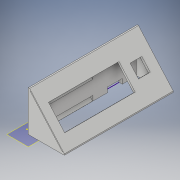
# Autodesk Inventor part: Suport - pantalla i potenciometre
Saved by Autodesk Inventor 2019 (Build 230136000, 136)
## iProperties
Created: 2018-08-18
Part Number: Suport - pantalla i potenciometre
Material: Genérico
Document SubType Name: Modeling
Designer: Albert Garangou Culebras
Density: 1 g/cm^3
Appearance: Valor por defecto
Author: Albert Garangou Culebras
Autodesk Inventor part; units mm, degrees
ref_plane "YZ Plane" through (0, 0, 0) normal (1, 0, 0) x (0, 1, 0)
ref_plane "XZ Plane" through (0, 0, 0) normal (0, 1, 0) x (-1, 0, 0)
ref_plane "XY Plane" through (0, 0, 0) normal (0, 0, 1) x (1, 0, 0)
sketch "Boceto3" plane through (0, 0, 0) normal (0, 0, 1) x (1, 0, 0)
  line L0 (40, 0) -> (37, 0)
  line L1 (0, 0) -> (0, 45)
  line L2 (0, 45) -> (3, 45)
  line L3 (40, 0) -> (40, 3)
  line L4 (40, 3) -> (3, 45)
  line L5 (0, 0) -> (40, 0)
  dimension "d3" = 3
  dimension "d4" = 45
  dimension "d5" = 3
  dimension "d6" = 3
  constraints: 12 end point, 2 horizontal, 2 vertical, 1 perpendicular
  measures "d3" distance of L0.start L0.end
  measures "d4" distance of L1.start L1.end
  measures "d5" distance of L1.end L2.end
  measures "d6" distance of L0.start L3.end
extrude "Extrusión1" add sketch "Boceto3" against normal blind 98.2
sketch "Boceto4" plane through (0, 0, 0) normal (0, 0, 1) x (1, 0, 0)
  line L0 (3.315362, 41.620064) -> (2, 43)
  line L1 (3.315362, 41.620064) -> (38, 2)
  line L2 (38, 2) -> (2, 2)
  line L3 (2, 2) -> (2, 43)
  point P0 (0, 45)
  constraints: 8 end point, 1 horizontal
extrude "Extrusión2" cut sketch "Boceto4" against normal blind 210.55
sketch "Boceto6" plane through (0, 0, 0) normal (0, 0, 1) x (1, 0, 0)
  line L0 (1.039471, 0.999221) -> (39.039471, 0.999221)
  line L1 (39.039471, 1.000307) -> (39.039471, 1.999307)
  line L2 (39.039471, 0.999221) -> (39.039471, 1.999307)
  line L3 (39.039471, 1.999307) -> (3, 44.000307)
  line L4 (2.880008, 44.000307) -> (1.000008, 44.000307)
  line L5 (3, 44.000307) -> (1.000008, 44.000307)
  line L6 (1.000008, 1.000307) -> (39.039471, 1.000307)
  line L7 (1.000008, 44.000307) -> (1.000008, 1.000307)
  point P0 (0, 0)
  constraints: 10 end point, 2 perpendicular, 1 horizontal, 1 parallel
extrude "Extrusión3" add sketch "Boceto6" against normal blind 2
sketch "Boceto7" plane through (0, 0, -98.2) normal (0, 0, -1) x (-1, 0, 0)
  line L0 (-1.000008, 1.000307) -> (-39.039471, 1.000307)
  line L1 (-1.000008, 1.000307) -> (-39.039471, 1.000307)
  line L2 (-39.039471, 1.000307) -> (-39.039471, 2)
  line L3 (-39.039471, 1.999307) -> (-2.880008, 44.000307)
  line L4 (-39.039471, 2) -> (-2.880008, 44.000307)
  line L5 (-2.880008, 44.000307) -> (-1.000008, 44.000307)
  line L6 (-1.000008, 44.000307) -> (-1.000008, 1.000307)
  line L7 (-2.880008, 44.000307) -> (6.906678, 55.367839)
  line L8 (6.906678, 55.367839) -> (10.168907, 59.157016)
  line L9 (10.168907, 59.157016) -> (10.168907, 0)
  line L10 (10.168907, 0) -> (0, 0)
  dimension "d68" = 15
  dimension "d70" = 5
  constraints: 17 end point, 2 perpendicular, 2 vertical, 1 collinear
  measures "d68" distance of L3.end L7.end
  measures "d70" distance of L7.end L8.end
extrude "Extrusión4" add sketch "Boceto7" against normal blind 2
sketch "Boceto10" plane through (0, 0, -96.2) normal (0, 0, 1) x (1, 0, 0)
  line L0 (20.169084, 1.000307) -> (21.669084, 1.000307)
  line L1 (39.039471, 1.000307) -> (1.000008, 1.000307)
  line L2 (21.669084, 1.000307) -> (21.669084, 22.175869)
  line L3 (2.880008, 44.000307) -> (39.039471, 1.999307)
  line L4 (21.669084, 22.175869) -> (20.169084, 23.918193)
  line L5 (20.169084, 23.918193) -> (20.169084, 1.000307)
  point P0 (0, 0)
  dimension "d49" = 1.5
  constraints: 8 end point, 2 point on line, 1 collinear, 1 parallel, 1 vertical
  measures "d49" distance of L0.start L0.end
extrude "Extrusión7" add sketch "Boceto10" along normal blind 96
sketch "Boceto15" plane through (0, 0, -98.2) normal (0, 0, -1) x (-1, 0, 0)
  line L0 (-3, 45) -> (-40, 3)
  line L1 (-20.392682, 25.256955) -> (-7.172072, 40.264135)
  line L2 (-7.172072, 40.264135) -> (-7.172072, 0)
  line L3 (-20.169084, 1.000307) -> (-1.000008, 1.000307)
  line L4 (-7.172072, 40.264135) -> (-3, 45)
  line L5 (0, 45) -> (-3, 45)
  line L6 (0, 0) -> (0, 45)
  line L7 (0, 45) -> (0, 0)
  line L8 (0, 0) -> (-7.172072, 0)
  line L9 (-40, 0) -> (0, 0)
  dimension "d71" = 20
  constraints: 12 end point, 3 collinear, 2 point on line, 1 horizontal, 1 perpendicular
  measures "d71" distance of L1.start L1.end
extrude "Extrusión9" cut sketch "Boceto15" against normal blind 617.4
sketch "Boceto16" plane through (0, 0, -96.2) normal (0, 0, 1) x (1, 0, 0)
  line L0 (7.172072, 0.999997) -> (8.672072, 1.000307)
  line L1 (20.169084, 1.000307) -> (7.172072, 1.000307)
  line L2 (8.672072, 1.000307) -> (8.672072, 37.27254)
  line L3 (7.172072, 39.014864) -> (20.169084, 23.918193)
  line L4 (8.672072, 37.27254) -> (7.172072, 39.014864)
  line L5 (7.172072, 39.014864) -> (7.172072, 0.999997)
  point P0 (0, 0)
  dimension "d74" = 1.5
  constraints: 8 end point, 1 collinear, 1 parallel, 1 perpendicular, 1 point on line
  measures "d74" distance of L0.start L0.end
extrude "Extrusión10" add sketch "Boceto16" along normal blind 95.4
sketch "Boceto17" plane through (0, 0, 0) normal (0, 0, 1) x (1, 0, 0)
  line L0 (20.169084, 1.000307) -> (8.672072, 1.000307)
  line L1 (8.672072, 35.501126) -> (8.672072, 2)
  line L2 (8.672072, 1.000307) -> (8.672072, 37.27254)
  line L3 (39.039471, 1.999307) -> (21.669084, 22.175869)
  line L4 (8.672072, 37.27254) -> (39.039471, 1.999307)
  line L5 (39.039471, 1.999307) -> (39.039471, 1.000307)
  line L6 (39.039471, 1.000307) -> (8.672072, 1.000307)
  line L7 (40, 0) -> (7.172072, 0)
  point P0 (0, 0)
  constraints: 8 end point, 2 collinear, 2 parallel
extrude "Extrusión11" cut sketch "Boceto17" against normal blind 235.6
sketch "Boceto21" plane through (40, 3, 0) normal (0.750359, 0.6610305, 0) x (0, 0, -1)
  line L0 (5, 24.190145) -> (5, 36.190145)
  line L1 (5, 36.190145) -> (5, 12.190145)
  line L2 (76, 36.190145) -> (5, 36.190145)
  line L3 (85, 24.190145) -> (85, 18.190145)
  line L4 (85, 18.190145) -> (91, 18.190145)
  line L5 (91, 18.190145) -> (97, 18.190145)
  line L6 (97, 18.190145) -> (97, 30.190145)
  line L7 (97, 30.190145) -> (85, 30.190145)
  line L8 (85, 30.190145) -> (85, 24.190145)
  line L9 (76, 24.190145) -> (81, 24.190145)
  line L10 (81, 24.190145) -> (85, 24.190145)
  line L11 (76, 36.190145) -> (77, 36.190145)
  line L12 (77, 36.190145) -> (77, 12.190145)
  line L13 (77, 12.190145) -> (76, 12.190145)
  line L14 (77, 12.190145) -> (77, 11.190145)
  line L15 (77, 11.190145) -> (5, 11.190145)
  line L16 (5, 11.190145) -> (5, 12.190145)
  point P0 (0, 24.190145)
  dimension "d114" = 5
  dimension "d176" = 1
  dimension "d177" = 1
  constraints: 34 end point, 7 perpendicular, 3 horizontal, 3 point on line, 1 vertical
  measures "d114" distance of L9.end L9.start
  measures "d176" distance of L2.start L11.end
  measures "d177" distance of L12.end L14.end
extrude "Extrusión13" cut sketch "Boceto21" against normal blind 1.5
sketch "Boceto22" plane through (0, 0, 0) normal (0, 0, 1) x (1, 0, 0)
  line L0 (8.672072, 1.000307) -> (39.039471, 1.000307)
  line L1 (8.672072, 1.000307) -> (39.039471, 1.000307)
  line L2 (39.039471, 1.000307) -> (39.039471, 2)
  line L3 (39.039471, 2) -> (8.672072, 37)
  line L4 (8.672072, 37.27254) -> (8.672072, 1.000307)
  line L5 (8.672072, 37) -> (8.672072, 1.000307)
  line L6 (7.172072, 0) -> (7.172072, 40.264135)
  line L7 (7.172072, 40.264135) -> (7.172072, 0)
  line L8 (40, 3) -> (40, 0)
  line L9 (7.172072, 0) -> (40, 0)
  line L10 (40, 0) -> (40, 3)
  line L11 (40, 3) -> (7.172072, 40.264135)
  line L12 (7.172072, 40.264135) -> (40, 3)
  point P0 (0, 0)
  constraints: 16 end point, 3 collinear, 3 perpendicular, 1 horizontal
extrude "Extrusión14" add sketch "Boceto22" along normal blind 2
sketch "Boceto24" plane through (0, 0, 2) normal (0, 0, 1) x (1, 0, 0)
  line L0 (8.672072, 1.000307) -> (8.672072, 37)
  line L1 (39.039471, 1.000307) -> (8.672072, 1.000307)
  line L2 (8.672072, 1.000307) -> (39.039471, 1.000307)
  line L3 (39.039471, 1.000307) -> (39.039471, 2)
  line L4 (39.039471, 2) -> (8.672072, 37)
  line L5 (8.672072, 37) -> (8.672072, 1.000307)
  point P0 (0, 0)
  constraints: 8 end point, 1 collinear, 1 parallel, 1 perpendicular
extrude "Extrusión15" add sketch "Boceto24" against normal blind 2
sketch "Boceto25" plane through (0, 0, -98.2) normal (0, 0, -1) x (-1, 0, 0)
  line L0 (-8.672072, 1.000307) -> (-8.672072, 37.27254)
  line L1 (-8.672072, 1.000307) -> (-8.672072, 37.27254)
  line L2 (-8.672072, 37.27254) -> (-39, 2)
  line L3 (-39, 2) -> (-39, 1.000307)
  line L4 (-39, 1.000307) -> (-8.672072, 1.000307)
  line L5 (-7.172072, 0) -> (-40, 0)
  line L6 (-7.172072, 40) -> (-7.172072, 0)
  line L7 (-40, 0) -> (-7.172072, 0)
  line L8 (-40, 0) -> (-40, 2.859817)
  line L9 (-7.172072, 0) -> (-7.172072, 40.264135)
  line L10 (-40, 2.859817) -> (-7.172072, 40.264135)
  point P0 (0, 0)
  constraints: 16 end point, 2 parallel, 2 vertical, 1 collinear, 1 perpendicular
extrude "Extrusión16" add sketch "Boceto25" along normal blind 7
sketch "Boceto27" plane through (0, 0, -105.2) normal (0, 0, -1) x (-1, 0, 0)
  line L0 (-8.672072, 1.000307) -> (-39.039471, 1.000307)
  line L1 (-8.672072, 1.000307) -> (-39.039471, 1.000307)
  line L2 (-39.039471, 1.000307) -> (-39.039471, 1.999307)
  line L3 (-8.672072, 1.000307) -> (-8.672072, 37.27254)
  line L4 (-39.039471, 1.999307) -> (-8.672072, 37.27254)
  line L5 (-8.672072, 37.27254) -> (-8.672072, 1.000307)
  point P0 (0, 0)
  constraints: 8 end point, 2 collinear, 1 perpendicular
extrude "Extrusión17" add sketch "Boceto27" against normal blind 2
sketch "Boceto28" plane through (7.172072, 0, 2) normal (0, -1, 0) x (1, 0, 0)
  line L0 (0, 0) -> (0, -107.2)
  line L1 (32.827928, 0) -> (32.827928, -107.2)
  line L2 (0, 0) -> (32.827928, 0)
  line L3 (32.827928, 0) -> (32.827928, -107.2)
  line L4 (32.827928, -107.2) -> (0, -107.2)
  line L5 (0, -107.2) -> (0, 0)
  point P0 (-7.172072, -2)
  constraints: 8 end point, 2 parallel, 1 horizontal, 1 perpendicular
extrude "Extrusión18" add sketch "Boceto28" along normal blind 2
sketch "Boceto29" plane through (7.172072, 40.264135, -98.2) normal (-1, 0, 0) x (0, 0, 1)
  line L0 (0, 0) -> (-7, 0)
  line L1 (100.2, -37.264135) -> (100.2, -42.264135)
  line L2 (-7, 0) -> (100.2, 0)
  line L3 (100.2, 0) -> (100.2, -42.264135)
  line L4 (100.2, -42.264135) -> (-7, -42.264135)
  line L5 (-7, -42.264135) -> (-7, 0)
  point P0 (98.2, -40.264135)
  constraints: 8 end point, 2 parallel, 1 horizontal, 1 perpendicular
extrude "Extrusión19" add sketch "Boceto29" along normal blind 2
sketch "Boceto30" plane through (0, 0, -105.2) normal (0, 0, -1) x (-1, 0, 0)
  line L0 (-7.172072, 40.264135) -> (-5.172072, 40.264135)
  line L1 (-5.172072, 40.264135) -> (-5.172072, -2)
  line L2 (-5.172072, 40.264135) -> (-5.172072, -2)
  line L3 (-40, -2) -> (-5.172072, -2)
  line L4 (-5.172072, -2) -> (-40, -2)
  line L5 (-40, 2.859817) -> (-40, -2)
  line L6 (-40, -2) -> (-40, 2.859817)
  line L7 (-40, 2.859817) -> (-7.172072, 40.264135)
  line L8 (-7.172072, 40.264135) -> (-5.172072, 40.264135)
  point P0 (0, 0)
  constraints: 12 end point, 3 collinear, 1 horizontal, 1 perpendicular
extrude "Extrusión20" add sketch "Boceto30" along normal blind 2
sketch "Boceto31" plane through (0, 0, 2) normal (0, 0, 1) x (1, 0, 0)
  line L0 (5.172072, -2) -> (5.172072, 40.264135)
  line L1 (5.172072, 40.26431) -> (5.172072, -2)
  line L2 (40, -2) -> (5.172072, -2)
  line L3 (5.172072, -2) -> (40, -2)
  line L4 (40, 2.859817) -> (40, -2)
  line L5 (40, -2) -> (40, 2.859817)
  line L6 (40, 2.859817) -> (7.172072, 40.264135)
  line L7 (7.172072, 40.264135) -> (40, 2.859817)
  line L8 (7.172072, 40.264135) -> (5.172072, 40.264135)
  point P0 (0, 0)
  constraints: 11 end point, 3 collinear, 1 horizontal
extrude "Extrusión21" add sketch "Boceto31" along normal blind 2
sketch "Boceto32" plane through (40, 3, 2) normal (0.750359, 0.6610305, 0) x (0, 0, -1)
  line L0 (-2, 49.661742) -> (-2, 0)
  line L1 (-2, 0) -> (109.2, 0)
  line L2 (109.2, -3.751795) -> (109.2, 19.270529)
  line L3 (100.2, -0.105188) -> (109.2, -0.105188)
  line L4 (109.2, 49.661742) -> (109.2, -0.105188)
  line L5 (109.2, 49.661742) -> (-2, 49.661742)
  line L6 (-2, 50.983803) -> (-2, 19.270529)
  line L7 (7, 11.190145) -> (7, 36.190145)
  line L8 (7, 36.190145) -> (7, 12.190145)
  line L9 (78, 36.190145) -> (7, 36.190145)
  line L10 (87, 30.190145) -> (99, 30.190145)
  line L11 (87, 18.190145) -> (87, 30.190145)
  line L12 (87, 30.190145) -> (87, 18.190145)
  line L13 (99, 30.190145) -> (99, 18.190145)
  line L14 (87, 18.190145) -> (99, 18.190145)
  line L15 (99, 18.190145) -> (99, 30.190145)
  line L16 (100.2, 49.661742) -> (109.2, 49.661742)
  line L17 (109.2, 49.661742) -> (109.2, -0.105188)
  line L18 (-2, -3.751795) -> (-2, -0.105188)
  line L19 (109.2, -0.105188) -> (-2, -0.105188)
  line L20 (-2, -0.105188) -> (-2, 49.661742)
  line L21 (109.2, 49.661742) -> (-2, 49.661742)
  line L22 (87, 30.190145) -> (99, 30.190145)
  line L23 (7, 12.190145) -> (7, 11.190145)
  line L24 (7, 11.190145) -> (79, 11.190145)
  line L25 (79, 11.190145) -> (79, 36.190145)
  line L26 (79, 36.190145) -> (78, 36.190145)
  point P0 (2, 24.190145)
  dimension "d174" = 1
  dimension "d175" = 72
  constraints: 36 end point, 7 collinear, 6 perpendicular, 2 point on line, 2 vertical, 1 horizontal
  measures "d174" distance of L8.end L7.start
  measures "d175" distance of L7.start L24.end
extrude "Extrusión22" add sketch "Boceto32" along normal blind 1
sketch "Boceto33" plane through (40.750359, 3.661031, 2) normal (0.750359, 0.6610305, 0) x (0, 0, -1)
  line L0 (87, 30.190145) -> (87, 18.190145)
  line L1 (87, 30.190145) -> (99, 30.190145)
  line L2 (87, 30.190145) -> (99, 30.190145)
  line L3 (99, 30.190145) -> (99, 18.133841)
  line L4 (100.2, -0.105188) -> (100.2, 49.661742)
  line L5 (99, 18.133841) -> (87, 18.133841)
  line L6 (87, 30.190145) -> (87, 34.190145)
  line L7 (87, 34.190145) -> (83, 34.190145)
  line L8 (99, 18.190145) -> (99, 14.190145)
  line L9 (99, 14.190145) -> (103, 14.190145)
  line L10 (83, 34.190145) -> (103, 34.190145)
  line L11 (103, 34.190145) -> (103, 14.190145)
  line L12 (103, 14.190145) -> (83, 14.190145)
  line L13 (83, 14.190145) -> (83, 34.190145)
  point P0 (2, 24.190145)
  dimension "d126" = 4
  dimension "d127" = 4
  dimension "d129" = 4
  dimension "d130" = 4
  constraints: 22 end point, 4 perpendicular, 3 parallel, 2 horizontal, 2 vertical
  measures "d126" distance of L0.start L6.end
  measures "d127" distance of L6.end L7.end
  measures "d129" distance of L8.start L8.end
  measures "d130" distance of L8.end L9.end
extrude "Extrusión23" add sketch "Boceto33" against normal blind 2.5
sketch "Boceto34" plane through (40.750359, 3.661031, 2) normal (0.750359, 0.6610305, 0) x (0, 0, -1)
  line L0 (99, 18.190145) -> (99, 30.190145)
  line L1 (99, 18.190145) -> (87, 18.190145)
  line L2 (87, 18.190145) -> (87, 30.190145)
  line L3 (99, 30.190145) -> (99, 18.190145)
  line L4 (99, 30.190145) -> (99, 18.190145)
  line L5 (87, 18.190145) -> (99, 18.190145)
  line L6 (99, 30.190145) -> (99, 31.190145)
  line L7 (99, 31.190145) -> (87, 31.190145)
  line L8 (87, 31.190145) -> (87, 30.190145)
  point P0 (2, 24.190145)
  point P1 (83, 34.190145)
  dimension "d173" = 1
  constraints: 18 end point, 3 perpendicular, 1 collinear, 1 point on line
  measures "d173" distance of L0.end L6.end
extrude "Extrusión24" cut sketch "Boceto34" against normal blind 6
sketch "Boceto35" plane through (40.069532, 2.921072, 4) normal (0, 0, 1) x (0.750359, 0.6610305, 0)
  line L0 (0, 49.76693) -> (1, 49.76693)
  line L1 (1, 49.76693) -> (0, 49.76693)
  line L2 (0, 49.76693) -> (0, 0)
  line L3 (0, 0) -> (1, 0)
  line L4 (0, 0) -> (1, 0)
  line L5 (1, 0) -> (1, 49.76693)
  point P0 (-31.997451, 24.295332)
  constraints: 8 end point, 3 perpendicular, 1 horizontal
extrude "Extrusión25" cut sketch "Boceto35" against normal blind 0.0001
sketch "Boceto36" plane through (0, 0, 4) normal (0, 0, 1) x (1, 0, 0)
  line L0 (5.172072, 40.264135) -> (7.172072, 40.264135)
  line L1 (7.172072, 40.264135) -> (40, 2.859817)
  line L2 (5.172072, 40.264135) -> (7.172072, 40.264135)
  line L3 (7.172072, 40.264135) -> (7.922431, 40.925165)
  line L4 (7.172072, 40.264135) -> (7.922431, 40.925165)
  line L5 (7.922431, 40.925165) -> (6.60037, 42.425883)
  line L6 (6.60037, 42.425883) -> (5.172072, 42.425883)
  line L7 (5.172072, -2) -> (5.172072, 40.264135)
  line L8 (5.172072, 42.425883) -> (5.172072, 40.264135)
  point P0 (0, 0)
  dimension "d140" = 2
  constraints: 10 end point, 2 perpendicular, 1 collinear, 1 horizontal, 1 parallel
  measures "d140" distance of L3.end L5.end
extrude "Extrusión26" add sketch "Boceto36" against normal blind 111.22
sketch "Boceto37" plane through (0, 0, 4) normal (0, 0, 1) x (1, 0, 0)
  line L0 (40.069532, 2.921072) -> (7.172072, 40.264135)
  line L1 (40.069532, 2.921072) -> (39.994609, 2.855068)
  line L2 (39.994609, 2.855068) -> (7.13461, 40.231133)
  line L3 (7.172072, 40.264135) -> (7.922431, 40.925165)
  line L4 (7.13461, 40.231133) -> (7.922431, 40.925165)
  line L5 (7.922431, 40.925165) -> (40.069532, 2.921072)
  point P0 (0, 0)
  constraints: 8 end point, 1 collinear, 1 perpendicular
extrude "Extrusión27" add sketch "Boceto37" against normal blind 2 contours L1 L2 L4 L0
sketch "Boceto38" plane through (0, 0, 4) normal (0, 0, 1) x (1, 0, 0)
  line L0 (40, 2.859817) -> (40, -2)
  line L1 (40, -2) -> (40, 2.859817)
  line L2 (40.069532, 2.921072) -> (40.819891, 3.582102)
  line L3 (40, 2.859817) -> (40.819891, 3.582102)
  line L4 (40, -2) -> (42, -2)
  line L5 (42, -2) -> (42, 2.242519)
  line L6 (42, 2.242519) -> (40.819891, 3.582102)
  point P0 (0, 0)
  constraints: 10 end point, 2 collinear, 1 perpendicular
extrude "Extrusión28" add sketch "Boceto38" against normal blind 111.25
sketch "Boceto39" plane through (0, 0, -107.2) normal (0, 0, -1) x (-1, 0, 0)
  line L0 (-40.069532, 2.921072) -> (-40.819891, 3.582102)
  line L1 (-40.069532, 2.921072) -> (-40, 2.859817)
  line L2 (-40.069532, 2.921072) -> (-7.172072, 40.264135)
  line L3 (-40, 2.859817) -> (-7.172072, 40.264135)
  line L4 (-7.172072, 40.264135) -> (-40.069532, 2.921072)
  line L5 (-40.069532, 2.921072) -> (-40, 2.859817)
  point P0 (0, 0)
  constraints: 8 end point, 2 collinear, 1 perpendicular
extrude "Extrusión29" add sketch "Boceto39" against normal blind 2
sketch "Boceto40" plane through (7.172072, -2, 2) normal (0, -1, 0) x (1, 0, 0)
  line L0 (7.786838, -16.048701) -> (16.767817, -16.048701) construction
  line L1 (16.767817, -16.048701) -> (16.767817, -19.096701) construction
  line L2 (16.767817, -19.096701) -> (7.786838, -19.096701) construction
  line L3 (7.786838, -19.096701) -> (7.786838, -16.048701) construction
  spline S0 degree 2 poles (12.542267, -20.275201) (12.542267, -20.729982) (12.196238, -21.426984) (11.909528, -21.654374) knots 0 0 0 1 2 2 2
  spline S1 degree 2 poles (11.909528, -21.654374) (11.563499, -21.921311) (10.777519, -22.148702) (10.154666, -22.148702) knots 0 0 0 1 2 2 2
  line L4 (10.154666, -22.148702) -> (8.404747, -22.148702)
  line L5 (8.404747, -22.148702) -> (8.404747, -16.048701)
  line L6 (8.404747, -16.048701) -> (10.021198, -16.048701)
  spline S2 degree 2 poles (10.021198, -16.048701) (10.67371, -16.048701) (11.326222, -16.132737) (11.622818, -16.295865) knots 0 0 0 1 2 2 2
  spline S3 degree 2 poles (11.622818, -16.295865) (11.954018, -16.46888) (12.255558, -17.037356) (12.255558, -17.422932) knots 0 0 0 1 2 2 2
  spline S4 degree 2 poles (12.255558, -17.422932) (12.255558, -17.852996) (11.800776, -18.535168) (11.400371, -18.727956) knots 0 0 0 1 2 2 2
  line L7 (11.400371, -18.727956) -> (11.400371, -18.757616)
  spline S5 degree 2 poles (11.400371, -18.757616) (11.944131, -18.905914) (12.542267, -19.691894) (12.542267, -20.275201) knots 0 0 0 1 2 2 2
  spline S6 degree 2 poles (11.696968, -20.309804) (11.696968, -19.963774) (11.499237, -19.51888) (11.20264, -19.360695) knots 0 0 0 1 2 2 2
  spline S7 degree 2 poles (11.20264, -19.360695) (11.009852, -19.26183) (10.555071, -19.20251) (10.134893, -19.20251) knots 0 0 0 1 2 2 2
  line L8 (10.134893, -19.20251) -> (9.215444, -19.20251)
  line L9 (9.215444, -19.20251) -> (9.215444, -21.456643)
  line L10 (9.215444, -21.456643) -> (9.872899, -21.456643)
  spline S8 degree 2 poles (9.872899, -21.456643) (10.406773, -21.456643) (11.019739, -21.357778) (11.257016, -21.199593) knots 0 0 0 1 2 2 2
  spline S9 degree 2 poles (11.257016, -21.199593) (11.484407, -21.036465) (11.696968, -20.631116) (11.696968, -20.309804) knots 0 0 0 1 2 2 2
  spline S10 degree 2 poles (11.410258, -17.536627) (11.410258, -17.319123) (11.261959, -16.992867) (11.098831, -16.898945) knots 0 0 0 1 2 2 2
  spline S11 degree 2 poles (11.098831, -16.898945) (10.9011, -16.790193) (10.421603, -16.74076) (9.991538, -16.74076) knots 0 0 0 1 2 2 2
  line L11 (9.991538, -16.74076) -> (9.215444, -16.74076)
  line L12 (9.215444, -16.74076) -> (9.215444, -18.525282)
  line L13 (9.215444, -18.525282) -> (10.134893, -18.525282)
  spline S12 degree 2 poles (10.134893, -18.525282) (10.515525, -18.525282) (10.876384, -18.446189) (11.069172, -18.322607) knots 0 0 0 1 2 2 2
  spline S13 degree 2 poles (11.069172, -18.322607) (11.257016, -18.203969) (11.410258, -17.823337) (11.410258, -17.536627) knots 0 0 0 1 2 2 2
  line L14 (12.690566, -22.148702) -> (14.746968, -16.048701)
  line L15 (14.746968, -16.048701) -> (15.745509, -16.048701)
  line L16 (15.745509, -16.048701) -> (17.801911, -22.148702)
  line L17 (17.801911, -22.148702) -> (16.946725, -22.148702)
  line L18 (16.946725, -22.148702) -> (16.393078, -20.443272)
  line L19 (16.393078, -20.443272) -> (14.064796, -20.443272)
  line L20 (14.064796, -20.443272) -> (13.511149, -22.148702)
  line L21 (13.511149, -22.148702) -> (12.690566, -22.148702)
  line L22 (16.170631, -19.751214) -> (15.226465, -16.879171)
  line L23 (15.226465, -16.879171) -> (14.287243, -19.751214)
  line L24 (14.287243, -19.751214) -> (16.170631, -19.751214)
  line L25 (20.505882, -22.148702) -> (18.142997, -22.148702)
  line L26 (18.142997, -22.148702) -> (18.142997, -21.525849)
  line L27 (18.142997, -21.525849) -> (18.919091, -21.525849)
  line L28 (18.919091, -21.525849) -> (18.919091, -16.671554)
  line L29 (18.919091, -16.671554) -> (18.142997, -16.671554)
  line L30 (18.142997, -16.671554) -> (18.142997, -16.048701)
  line L31 (18.142997, -16.048701) -> (20.505882, -16.048701)
  line L32 (20.505882, -16.048701) -> (20.505882, -16.671554)
  line L33 (20.505882, -16.671554) -> (19.729788, -16.671554)
  line L34 (19.729788, -16.671554) -> (19.729788, -21.525849)
  line L35 (19.729788, -21.525849) -> (20.505882, -21.525849)
  line L36 (20.505882, -21.525849) -> (20.505882, -22.148702)
  line L37 (25.725979, -22.148702) -> (24.796644, -22.148702)
  line L38 (24.796644, -22.148702) -> (23.313662, -19.716611)
  line L39 (23.313662, -19.716611) -> (21.80102, -22.148702)
  line L40 (21.80102, -22.148702) -> (20.92606, -22.148702)
  line L41 (20.92606, -22.148702) -> (22.868767, -19.093758)
  line L42 (22.868767, -19.093758) -> (20.985379, -16.048701)
  line L43 (20.985379, -16.048701) -> (21.914715, -16.048701)
  line L44 (21.914715, -16.048701) -> (23.368038, -18.436303)
  line L45 (23.368038, -18.436303) -> (24.85102, -16.048701)
  line L46 (24.85102, -16.048701) -> (25.725979, -16.048701)
  line L47 (25.725979, -16.048701) -> (23.817875, -19.054212)
  line L48 (23.817875, -19.054212) -> (25.725979, -22.148702)
  point P0 (-7.172072, -2)
  constraints: 2 other
extrude "Extrusión30" cut sketch "Boceto40" against normal blind 0.5
sketch "Boceto41" plane through (8.672072, 1.000307, 0) normal (0, 1, 0) x (1, 0, 0)
  circle A0 centre (15, 56) radius 1.6
  circle A1 centre (15, 23) radius 1.6
  point P0 (-8.672072, 0)
  dimension "d155" = 3.2
  dimension "d156" = 3.2
  constraints: 2 centre point
  measures "d155" diameter of A0
  measures "d156" diameter of A1
extrude "Extrusión31" cut sketch "Boceto41" against normal blind 65.25
sketch "Boceto42" plane through (5.172072, 40.264135, -98.2) normal (-1, 0, 0) x (0, 0, 1)
  line L0 (9.7, -39.263828) -> (9.7, -34.263828)
  line L1 (9.7, -34.263828) -> (24.7, -34.263828)
  line L2 (24.7, -34.263828) -> (24.7, -39.263828)
  line L3 (9.7, -39.263828) -> (24.7, -39.263828)
  line L4 (0, -39.263828) -> (98.2, -39.263828)
  point P0 (98.2, -40.264135)
  point P1 (17.2, -27.607978)
  constraints: 8 end point, 2 perpendicular, 1 collinear
extrude "Extrusión32" cut sketch "Boceto42" against normal blind 6.25
sketch "Boceto43" plane through (5.172072, 40.264135, -98.2) normal (-1, 0, 0) x (0, 0, 1)
  line L0 (21.2, -10.748812) -> (93.2, -10.748812)
  line L1 (93.2, -10.748812) -> (40, -10.748812)
  line L2 (40, -10.748812) -> (40, -15.748812)
  line L3 (40, -15.748812) -> (93.2, -15.748812)
  line L4 (93.2, -15.748812) -> (93.2, -10.748812)
  line L5 (93.2, -35) -> (40, -35)
  line L6 (40, -35) -> (40, -30)
  line L7 (40, -30) -> (93.2, -30)
  line L8 (93.2, -30) -> (93.2, -35)
  line L9 (103, -15.748812) -> (118.556349, -15.748812) construction
  point P0 (98.2, -40.264135)
  point P1 (22.2, -10.748812)
  dimension "d164" = 5
  dimension "d165" = 5
  constraints: 18 end point, 4 parallel, 3 horizontal, 2 perpendicular
  measures "d164" distance of L2.end L1.end
  measures "d165" distance of L5.end L6.end
sketch "Boceto44" plane through (0, 0, 4) normal (0, 0, 1) x (1, 0, 0)
  line L0 (5.172072, -2) -> (5.172072, 40.264135)
  line L1 (5.172072, 19.132067) -> (16, 6.227845)
  line L2 (5.172072, 19.132067) -> (22.017338, 19.132067) construction
  point P0 (0, 0)
  dimension "d167" = 50
  constraints: 4 end point, 1 equal length, 1 horizontal, 1 midpoint
  measures "d167" angle of L1 L2
sweep "Barrido1" cut profiles "Boceto43" path "Boceto44" keep normal constant yes path curves L1
sketch "Boceto45" plane through (7.172072, -2, 2) normal (0, -1, 0) x (1, 0, 0)
  line L0 (4.095333, -60.2) -> (8.290831, -60.2)
  line L1 (8.290831, -7) -> (4.095333, -7)
  line L2 (8.290831, -7) -> (0, -7)
  line L3 (0, -7) -> (0, -60.2)
  line L4 (0, -60.2) -> (8.290831, -60.2)
  line L5 (8.290831, -60.2) -> (8.290831, -7)
  point P0 (-7.172072, -2)
  constraints: 12 end point, 3 parallel, 2 horizontal, 1 perpendicular
extrude "Extrusión33" add sketch "Boceto45" against normal blind 3
sketch "Boceto46" plane through (8.672072, 1.000307, 0) normal (0, 1, 0) x (1, 0, 0)
  line L0 (-3.5, 73.5) -> (-3.5, 88.5) projected
  line L1 (-3.5, 73.5) -> (-3.5, 88.5)
  point P0 (-8.672072, 0)
  constraints: 2 end point, 1 collinear
ref_plane "Plano de trabajo5" through (5.172072, 1.000307, 4) normal (0, -1, 0) x (1, 0, 0)
sketch "Boceto47" plane through (5.172072, 1.000307, 4) normal (0, -1, 0) x (1, 0, 0)
  line L0 (36.827928, 0) -> (36.827928, -111.25)
  line L1 (0, 0) -> (0, -111.22)
  line L2 (36.827928, -111.25) -> (0, -111.25)
  line L3 (0, -111.25) -> (0, 0)
  line L4 (0, 0) -> (36.827928, 0)
  line L5 (36.827928, 0) -> (36.827928, -111.25)
  point P0 (-5.172072, -4)
  constraints: 8 end point, 2 parallel, 1 horizontal, 1 perpendicular
extrude "Extrusión34" cut sketch "Boceto47" along normal blind 22.5
